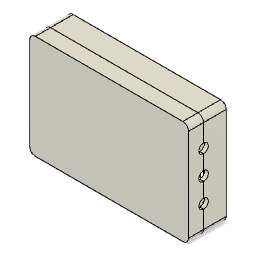
FanControlBox_v21 (Autodesk Fusion 360 design; units mm, degrees)
Autodesk Fusion 360 part; units mm, degrees
note: some values were not read from the file. Chosen so that the rebuilt part matches the saved one: which bodies a step acts on; which face or edge a step refers to. Set by a fixed rule: which sketch regions a step uses.
sketch "Sketch1" plane through (0, 0, 0) normal (0, 0, 1) x (1, 0, 0) in component "Box Base"
  line L0 (0, 85) -> (0, -85) construction
  line L1 (-107.0812, 0) -> (107.0812, 0) construction
  line L2 (0, 0) -> (-42, 0)
  line L3 (-42, 0) -> (-42, 27.5)
  line L4 (-42, 27.5) -> (0, 27.5)
  line L5 (0, 27.5) -> (0, 0)
  line L6 (0, 0) -> (-35.05, 0)
  line L7 (-35.05, 0) -> (-35.05, 25.05)
  line L8 (-35.05, 25.05) -> (0, 25.05)
  line L9 (0, 25.05) -> (0, 0)
  line L10 (0, 0) -> (-40, 0)
  line L11 (-40, 0) -> (-40, 25.5)
  line L12 (-40, 25.5) -> (0, 25.5)
  line L13 (0, 25.5) -> (0, 0)
  line L14 (0, 0) -> (-33.05, 0)
  line L15 (-33.05, 0) -> (-33.05, 23.05)
  line L16 (-33.05, 23.05) -> (0, 23.05)
  line L17 (0, 23.05) -> (0, 0)
  line L18 (-35.5, 27.5) -> (-35.5, 21)
  line L19 (-35.5, 21) -> (-42, 21)
  circle A0 centre (-38.5, 24) radius 1.25
  dimension "d5" = 42
  dimension "d6" = 27.5
  dimension "d10" = 25.05
  dimension "d11" = 35.05
  dimension "d12" = 2
  dimension "d13" = 2
  dimension "d15" = 2
  dimension "d16" = 2
  dimension "d81" = 0
  dimension "d82" = 0
  dimension "d83" = 0
  dimension "d84" = 0
  dimension "d171" = 3.5
  dimension "d172" = 3.5
  dimension "d183" = 0
  dimension "d184" = 0
  dimension "d185" = 0
  dimension "d186" = 0
  dimension "d199" = 6.5
  dimension "d200" = 6.5
  dimension "d249" = 0
  dimension "d250" = 0
  dimension "d251" = 0
  dimension "d252" = 0
  dimension "d259" = 2.5
  constraint vertical L0
  constraint perpendicular L0 L1
  constraint midpoint L2.start L1
  constraint midpoint L2.start L0
  constraint horizontal L2
  constraint vertical L3
  constraint horizontal L4
  constraint vertical L5
  constraint coincident L2.start L5.end
  constraint horizontal L6
  constraint vertical L7
  constraint horizontal L8
  constraint vertical L9
  constraint horizontal L10
  constraint vertical L11
  constraint horizontal L12
  constraint vertical L13
  constraint horizontal L14
  constraint vertical L15
  constraint horizontal L16
  constraint vertical L17
  constraint coincident L4 L18.start
  constraint perpendicular L4 L18
  constraint coincident L3 L19.end
  constraint perpendicular L3 L19
  measures "d5" distance of L0 L3
  measures "d6" distance of L1 L4
  measures "d10" distance of L1 L8
  measures "d11" distance of L5 L7
  measures "d12" distance of L4 L12
  measures "d13" distance of L3 L11
  measures "d15" distance of L8 L16
  measures "d16" distance of L7 L15
  measures "d171" distance of L3 A0.centre
  measures "d172" distance of L4 A0.centre
  measures "d199" distance of L3 L18
  measures "d200" distance of L4 L19
  measures "d259" diameter of A0
extrude "Extrude1" add sketch "Sketch1" along normal blind 1.5 contours L2 L5 L6 L9 L10 L13 L14 L15 L16 L17 | L2 L5 L6 L7 L8 L9 L10 L13 L15 L16 | L2 L5 L7 L8 L10 L11 L12 L13 L18 L19 | L2 L3 L11 L19 | L4 L5 L12 L18 | L3 L4 L11 L12 L18 L19 | L11 L12 L18 L19 | A0 makes body 1 in component "Box Base"
extrude "Extrude2" add sketch "Sketch1" along normal blind 8 contours L2 L3 L11 L19 | L4 L5 L12 L18 | L3 L4 L11 L12 L18 L19 | L11 L12 L18 L19 | A0 bodies 1 in component "Box Base"
extrude "Extrude4" add sketch "Sketch1" along normal blind 3 from surface at 1.5 contours L2 L5 L7 L8 L10 L11 L12 L13 L18 L19 bodies 1 in component "Box Base"
extrude "Extrude5" add sketch "Sketch1" along normal blind 1.5 from surface at 1.5 contours L2 L5 L6 L7 L8 L9 L10 L13 L15 L16 bodies 1 in component "Box Base"
extrude "Extrude6" cut sketch "Sketch1" against normal blind 4 from surface at 8 contours A0 bodies 1 in component "Box Base"
fillet "Fillet1" radius 3 1 edges at (-42, 27.5, 4) on bodies 1 in component "Box Base"
fillet "Fillet3" radius 0.5 1 edges at (-33.05, 23.05, 2.25) on bodies 1 in component "Box Base"
fillet "Fillet4" radius 2 1 edges at (-35.5, 21, 6.25) on bodies 1 in component "Box Base"
fillet "Fillet4" radius 0.5 2 edges at (-40, 21, 6.25) (-35.5, 25.5, 6.25) on bodies 1 in component "Box Base"
mirror "Mirror1" about plane through (0, 0, 0) normal (1, 0, 0) of bodies 1 makes body 2 in component "Box Base"
mirror "Mirror2" about plane through (0, 0, 0) normal (0, 1, 0) of bodies 1 2 makes body 3 at (-27, -9.1667, 0) makes body 4 at (27, -9.1667, 0) in component "Box Base"
combine "Combine1" operation add target body 1 tool bodies 2 4 3 in component "Box Base"
sketch "Sketch2" plane through (42, 0, 0) normal (1, 0, 0) x (0, 0, -1) in component "Box Base"
  line L0 (26.8483, 0) -> (-26.8483, 0) construction
  circle A0 centre (-8, 0) radius 2.5
  circle A1 centre (-8, 12.7) radius 2.5
  circle A2 centre (-8, -12.7) radius 2.5
  line L1 (-8, 24.5) -> (-8, -24.5)
  line L2 (0, -24.5) -> (0, 24.5)
  line L3 (-4.5, 25.05) -> (-4.5, -25.05)
  line L4 (0, 24.5) -> (-8, 24.5)
  line L5 (-8, -24.5) -> (0, -24.5)
  dimension "d43" = 5
  dimension "d44" = 5
  dimension "d45" = 5
  dimension "d143" = 12.7
  dimension "d144" = 12.7
  constraint midpoint origin L0
  constraint coincident L0 A0.centre
  constraint horizontal L0
  constraint coincident A1.centre L1
  constraint coincident A0.centre L1
  constraint coincident A2.centre L1
  measures "d43" diameter of A0
  measures "d44" diameter of A1
  measures "d45" diameter of A2
  measures "d143" distance of L0 A1.centre
  measures "d144" distance of L0 A2.centre
extrude "Extrude7" cut sketch "Sketch2" against normal blind 10 contours A0 L1 | A0 L1 | A1 L1 | A1 L1 | A2 L1 | A2 L1 bodies 1 in component "Box Base"
sketch "Sketch3" plane through (-42, 0, 0) normal (-1, 0, 0) x (0, 0, 1) in component "Box Base"
  line L0 (8, 24.5) -> (0, 24.5)
  line L1 (-35.9111, 0) -> (35.9111, 0) construction
  circle A0 centre (8, 2.54) radius 2.5
  circle A1 centre (8, -10.16) radius 2.5
  circle A2 centre (8, 12.7) radius 2.5
  line L2 (8, 24.5) -> (8, -24.5)
  line L3 (0, 24.5) -> (8, 24.5)
  line L4 (0, -24.5) -> (0, 24.5)
  line L5 (4.5, -25.05) -> (4.5, 25.05)
  line L6 (0, -24.5) -> (8, -24.5)
  dimension "d51" = 5
  dimension "d53" = 5
  dimension "d54" = 10.16
  dimension "d55" = 5
  dimension "d56" = 12.7
  dimension "d59" = 2.54
  constraint horizontal L1
  constraint midpoint origin L1
  constraint coincident A2.centre L2
  constraint coincident A0.centre L2
  constraint coincident A1.centre L2
  measures "d51" diameter of A0
  measures "d53" diameter of A1
  measures "d54" distance of L1 A1.centre
  measures "d55" diameter of A2
  measures "d56" distance of L1 A2.centre
  measures "d59" distance of L1 A0.centre
extrude "Extrude8" cut sketch "Sketch3" against normal blind 10 contours A2 L2 | A2 L2 | A0 L2 | A0 L2 | A1 L2 | A1 L2 bodies 1 in component "Box Base"
sketch "Sketch1 (2)" plane through (0, 0, 0) normal (0, 0, 1) x (1, 0, 0) in component "Box Lid"
  line L0 (0, 85) -> (0, -85) construction
  line L1 (-107.0812, 0) -> (107.0812, 0) construction
  line L2 (0, 0) -> (-42, 0)
  line L3 (-42, 0) -> (-42, 27.5)
  line L4 (0, 27.5) -> (0, 0)
  line L5 (0, 0) -> (-35.125, 0)
  line L6 (0, 25.125) -> (0, 0)
  line L7 (0, 0) -> (-40.5, 0)
  line L8 (0, 26) -> (0, 0)
  line L9 (0, 0) -> (-33.125, 0)
  line L10 (0, 23.125) -> (0, 0)
  circle A0 centre (-38.5, 24) radius 1
  line L11 (-35.5, 27.5) -> (-35.5, 23)
  line L12 (-37.5, 21) -> (-42, 21)
  circle A1 centre (-33.5, 23.5) radius 1.925
  line L13 (-40, 0) -> (-40, 21)
  line L14 (0, 25.5) -> (-35.5, 25.5)
  line L15 (-42, 27.5) -> (0, 27.5)
  line L16 (-31.575, 23.5) -> (-31.575, 25.5)
  arc A2 (-37.5, 21) -> (-35.5, 23) centre (-37.5, 23) ccw
  line L17 (-33.508, 21.575) -> (-36.0858, 21.5858)
  dimension "d5_1" = 42
  dimension "d32_1" = 2
  dimension "d81_1" = 0
  dimension "d82_1" = 0
  dimension "d83_1" = 0
  dimension "d84_1" = 0
  dimension "d175" = 3.5
  dimension "d187" = 0
  dimension "d188" = 0
  dimension "d189" = 0
  dimension "d190" = 0
  dimension "d202" = 6.5
  dimension "d228" = 3.85
  dimension "d237" = 2
  dimension "d238" = 27.5
  dimension "d239" = 2
  dimension "d240" = 6.5
  dimension "d241" = 3.5
  dimension "d242" = 2
  dimension "d243" = 2
  dimension "d253" = 0
  dimension "d254" = 0
  dimension "d255" = 0
  dimension "d256" = 0
  dimension "d257" = 2
  constraint vertical L0
  constraint perpendicular L0 L1
  constraint midpoint L2.start L1
  constraint midpoint L2.start L0
  constraint horizontal L2
  constraint vertical L3
  constraint vertical L4
  constraint coincident L2.start L4.end
  constraint horizontal L5
  constraint vertical L6
  constraint horizontal L7
  constraint vertical L8
  constraint horizontal L9
  constraint vertical L10
  constraint coincident L3 L12.end
  constraint perpendicular L3 L12
  constraint coincident L1 L13.start
  constraint coincident L12 L13.end
  constraint perpendicular L12 L13
  constraint coincident L4 L14.start
  constraint coincident L11 L14.end
  constraint perpendicular L11 L14
  constraint perpendicular L0 L15
  constraint coincident A1 L16.start
  constraint coincident L14 L16.end
  constraint tangent A1 L16
  constraint perpendicular L14 L16
  constraint tangent L11 A2
  constraint tangent L12 A2
  constraint coincident A1 L17.start
  constraint midpoint A2 L17.end
  constraint tangent A1 L17
  measures "d5_1" distance of L0 L3
  measures "d32_1" diameter of A0
  measures "d175" distance of L3 A0.centre
  measures "d202" distance of L3 L11
  measures "d228" diameter of A1
  measures "d237" distance of L3 L13
  measures "d238" distance of L1 L15
  measures "d239" distance of L14 L15
  measures "d240" distance of L12 L15
  measures "d241" distance of A0.centre L15
  measures "d242" distance of L11 A1.centre
  measures "d243" distance of A1.centre L14
  measures "d257" radius of A2
extrude "Extrude1'" add sketch "Sketch1 (2)" along normal blind 1.5 separate body contours L2 L4 L5 L6 L7 L8 L9 L10 L12 A1 L13 L14 L16 A2 L17 | L2 L3 L7 L12 L13 | L4 L8 L11 L14 L15 | L3 L11 L12 L15 A2 | L11 A1 L14 L16 A2 L17 | A1 | A0 makes body 5 in component "Box Lid"
extrude "Extrude2'" add sketch "Sketch1 (2)" along normal blind 12 contours L2 L3 L7 L12 L13 | L4 L8 L11 L14 L15 | L3 L11 L12 L15 A2 | A0 bodies 5 in component "Box Lid"
extrude "Extrude3" add sketch "Sketch1 (2)" along normal blind 12 contours L11 A1 L14 L16 A2 L17 | A1 bodies 5 in component "Box Lid"
extrude "Extrude12" add sketch "Sketch1 (2)" along normal blind 3.5 from surface at 12 contours A1 bodies 5 in component "Box Lid"
extrude "Extrude6'" cut sketch "Sketch1 (2)" against normal blind 12 from surface at 12 contours A0 bodies 5 in component "Box Lid"
chamfer "Chamfer4" distance 1.5 angle 45 1 edges at (-39.4323, 23.6384, 0) on bodies 5 in component "Box Lid"
fillet "Fillet1'" radius 3 1 edges at (-42, 27.5, 6) on bodies 5 in component "Box Lid"
fillet "Fillet8" radius 0.5 3 edges at (-40, 21, 6.75) (-31.575, 25.5, 6.75) (-36.0858, 21.5858, 6.75) on bodies 5 in component "Box Lid"
mirror "Mirror1'" about plane through (0, 0, 0) normal (1, 0, 0) of bodies 5 makes body 6 in component "Box Lid"
mirror "Mirror2'" about plane through (0, 0, 0) normal (0, 1, 0) of bodies 5 6 makes body 7 at (12.0825, -16.8051, 0) makes body 8 at (-12.0825, -16.8051, 0) in component "Box Lid"
combine "Combine1'" operation add target body 5 tool bodies 8 6 7 in component "Box Lid"
fillet "Fillet5" radius 0.5 1 faces at (-10.6274, -7.4856, 1.5) on bodies 5 in component "Box Lid"
sketch "Sketch2 (2)" plane through (42, 0, 0) normal (1, 0, 0) x (0, 0, -1) in component "Box Lid"
  line L0 (26.8483, 0) -> (-26.8483, 0) construction
  circle A0 centre (-12, 0) radius 2.5
  circle A1 centre (-12, 12.7) radius 2.5
  circle A2 centre (-12, -12.7) radius 2.5
  line L1 (-12, 24.5) -> (-12, -24.5)
  line L2 (0, -24.5) -> (0, 24.5)
  line L3 (0, 24.5) -> (-12, 24.5)
  line L4 (-12, -24.5) -> (0, -24.5)
  dimension "d43_1" = 5
  dimension "d44_1" = 5
  dimension "d45_1" = 5
  dimension "d143_1" = 12.7
  dimension "d144_1" = 12.7
  constraint midpoint origin L0
  constraint coincident L0 A0.centre
  constraint horizontal L0
  constraint coincident A1.centre L1
  constraint coincident A0.centre L1
  constraint coincident A2.centre L1
  measures "d43_1" diameter of A0
  measures "d44_1" diameter of A1
  measures "d45_1" diameter of A2
  measures "d143_1" distance of L0 A1.centre
  measures "d144_1" distance of L0 A2.centre
extrude "Extrude7'" cut sketch "Sketch2 (2)" against normal blind 10 contours A0 L1 | A0 L1 | A1 L1 | A1 L1 | A2 L1 | A2 L1 bodies 5 in component "Box Lid"
sketch "Sketch3 (2)" plane through (-42, 0, 0) normal (-1, 0, 0) x (0, 0, 1) in component "Box Lid"
  line L0 (-35.9111, 0) -> (35.9111, 0) construction
  circle A0 centre (12, -2.54) radius 2.5
  circle A1 centre (12, -12.7) radius 2.5
  circle A2 centre (12, 10.16) radius 2.5
  line L1 (0, 21) -> (0, -21) construction
  line L2 (12, 21) -> (12, -21) construction
  dimension "d51_1" = 5
  dimension "d53_1" = 5
  dimension "d54_1" = 12.7
  dimension "d55_1" = 5
  dimension "d56_1" = 10.16
  dimension "d146" = 2.54
  dimension "d248" = 12
  constraint horizontal L0
  constraint midpoint origin L0
  constraint vertical L1
  constraint midpoint origin L1
  constraint vertical L2
  constraint coincident A2.centre L2
  constraint coincident A0.centre L2
  constraint coincident A1.centre L2
  measures "d51_1" diameter of A0
  measures "d53_1" diameter of A1
  measures "d54_1" distance of L0 A1.centre
  measures "d55_1" diameter of A2
  measures "d56_1" distance of L0 A2.centre
  measures "d146" distance of L0 A0.centre
  measures "d248" distance of L1 L2
extrude "Extrude8'" cut sketch "Sketch3 (2)" against normal blind 10 bodies 5 in component "Box Lid"
sketch "Sketch4" plane through (0, 0, 0) normal (0, 0, -1) x (-1, 0, 0) in component "Box Lid"
  line L0 (42, -24.5) -> (42, 24.5)
  line L1 (-1.5, 20) -> (-1.5, 5)
  arc A0 (-1.5, 5) -> (1.5, 5) centre (0, 5) ccw
  line L2 (1.5, 5) -> (1.5, 20)
  arc A1 (1.5, 20) -> (-1.5, 20) centre (0, 20) ccw
  line L3 (0, 20) -> (0, 5) construction
  line L4 (-60.5, 0) -> (60.5, 0) construction
  line L5 (0, 40) -> (0, -40) construction
  line L6 (-42, 24.5) -> (-42, -24.5)
  line L7 (39, 27.5) -> (-39, 27.5)
  line L8 (-39, -27.5) -> (39, -27.5)
  arc A2 (42, 24.5) -> (39, 27.5) centre (39, 24.5) ccw
  arc A3 (-39, 27.5) -> (-42, 24.5) centre (-39, 24.5) ccw
  arc A4 (-42, -24.5) -> (-39, -27.5) centre (-39, -24.5) ccw
  arc A5 (39, -27.5) -> (42, -24.5) centre (39, -24.5) ccw
  circle A6 centre (-38.5, -24) radius 2.5
  circle A7 centre (-38.5, 24) radius 2.5
  circle A8 centre (38.5, -24) radius 2.5
  circle A9 centre (38.5, 24) radius 2.5
  dimension "d208" = 3
  dimension "d209" = 15
  dimension "d210" = 5
  constraint tangent L1 A0
  constraint tangent A0 L2
  constraint parallel L1 L2
  constraint tangent L2 A1
  constraint tangent L1 A1
  constraint vertical L3
  constraint horizontal L4
  constraint vertical L5
  constraint midpoint origin L5
  constraint midpoint origin L4
  constraint coincident A1.centre L5
  measures "d208" distance of L1 L2
  measures "d209" distance of A1.centre A0.centre
  measures "d210" distance of A0.centre L4
extrude "Extrude10" cut sketch "Sketch4" against normal through all contours L1 A0 L2 A1 bodies 5 in component "Box Lid"
pattern_linear "R-Pattern1" count 9 spacing 7.5 along (-1, 0, 0) both ways of "Extrude10" in component "Box Lid"
mirror "Mirror3" about plane through (0, 0, 0) normal (0, 1, 0) of "Extrude10", "R-Pattern1" in component "Box Lid"
component "Box Base" placed x (1, 0, 0) y (0, -1, 0) z (0, 0, -1) at (0, 0, 20)
component "Box Lid" placed x (1, 0, 0) y (0, 1, 0) z (0, 0, 1) at (0, 0, 0)
equation "Width = 55 mm"
equation "Length = 84 mm"
equation "Height = 20 mm"
equation "Wall = 1.5 mm"
equation "d5 = Length / 2"
equation "d6 = Width / 2"
equation "Wpcb = 50.1 mm"
equation "Lpcb = 70.1 mm"
equation "Tpcb = 1.5 mm"
equation "d10 = Wpcb / 2"
equation "d11 = Lpcb / 2"
equation "d12 = Side"
equation "d13 = Side"
equation "Lip = 2 mm"
equation "d15 = Lip"
equation "d16 = Lip"
equation "Corner = 6.5 mm"
equation "d20 = Wall"
equation "d22 = BaseHeight"
equation "d26 = 2 * Tpcb"
equation "d28 = Tpcb"
equation "d54 = ( 4 * 2.54 ) * 1 mm"
equation "d56 = ( 5 * 2.54 ) * 1 mm"
equation "Depth = Height - Wall - 2 * Tpcb"
equation "BaseHeight = 8 mm"
equation "d143 = ( 5 * 2.54 ) * 1 mm"
equation "d144 = ( 5 * 2.54 ) * 1 mm"
equation "d5_1 = Length / 2"
equation "d20_1 = Wall"
equation "d22_1 = LidHeight"
equation "d24_1 = LidHeight"
equation "d34_1 = -LidHeight"
equation "d54_1 = ( 5 * 2.54 ) * 1 mm"
equation "d56_1 = ( 4 * 2.54 ) * 1 mm"
equation "d143_1 = ( 5 * 2.54 ) * 1 mm"
equation "d144_1 = ( 5 * 2.54 ) * 1 mm"
equation "LidHeight = Height - BaseHeight"
equation "d171 = CornerHole"
equation "d172 = CornerHole"
equation "d175 = CornerHole"
equation "d199 = Corner"
equation "d200 = Corner"
equation "CornerHole = 3.5 mm"
equation "d202 = Corner"
equation "d226 = BaseHeight - Wall - 2 * Tpcb"
equation "Side = 2 mm"
equation "d237 = Side"
equation "d238 = Width / 2"
equation "d239 = Side"
equation "d240 = Corner"
equation "d241 = CornerHole"
equation "d248 = LidHeight"
